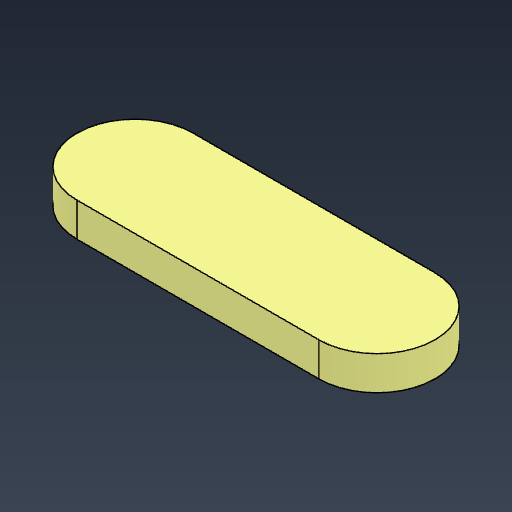
# Autodesk Inventor part: Dribblerdaempfer Unten V2
Saved by Autodesk Inventor 2023.1 (Build 271208000, 208)
## iProperties
Part Number: Dribblerdaempfer Unten V2
Material: Gummi, Silikon
Document SubType Name: Modeling
Designer: rYan
Density: 1.25 g/cm^3
Appearance: Gummi - Schwarz
Mass: 0.126032 g
Surface Area: 3.04725 cm^2
Volume: 0.100826 cm^3
Author: rYan
Autodesk Inventor part; units mm, degrees
ref_plane "YZ Plane" through (0, 0, 0) normal (1, 0, 0) x (0, 1, 0)
ref_plane "XZ Plane" through (0, 0, 0) normal (0, 1, 0) x (-1, 0, 0)
ref_plane "XY Plane" through (0, 0, 0) normal (0, 0, 1) x (1, 0, 0)
sketch "Skizze1" plane through (0, 0, 0) normal (0, 1, 0) x (-1, 0, 0)
  line L0 (0, 0) -> (14.8, 0)
  line L1 (14.8, 0) -> (14.8, 1.4)
  line L2 (0, 1.4) -> (0, 0)
  line L3 (14.8, 1.4) -> (11.5, 1.4)
  line L4 (11.5, 1.4) -> (11.5, 1.4)
  line L5 (11.1, 1.4) -> (11.1, 1.4)
  line L6 (7.6, 1.4) -> (0, 1.4)
  line L7 (11.1, 1.4) -> (8, 1.4)
  line L8 (8, 1.4) -> (8, 1.4)
  line L9 (7.6, 1.4) -> (7.6, 1.4)
  line L10 (11.5, 1.4) -> (11.1, 1.4)
  line L11 (8, 1.4) -> (7.6, 1.4)
  line L12 (11.3, 1.4) -> (11.3, 0.8) construction
  line L13 (7.8, 1.4) -> (7.8, 0.8) construction
  dimension "d1" = 14.8
  dimension "d3" = 1.4
  dimension "d17" = 1.4
  dimension "d18" = 1.4
  dimension "d19" = 3.5
  dimension "d20" = 0.4
  dimension "d21" = 0.4
  dimension "d22" = 7
  dimension "d23" = 60
  dimension "d24" = 60
  constraints: 28 end point, 4 horizontal, 3 point on line, 2 equal length, 2 midpoint, 2 vertical, 1 perpendicular, 2 other
  measures "d1" distance of L0.start L0.end
  measures "d3" distance of L2.start L0.start
  measures "d17" distance between parallel lines of L10 L0
  measures "d18" distance between parallel lines of L11 L0
  measures "d19" distance between parallel lines of L1 L12
  measures "d20" distance of L4.end L5.start
  measures "d21" distance of L8.end L9.start
  measures "d22" distance between parallel lines of L13 L1
  measures "d23" angle of L5 L4
  measures "d24" angle of L9 L8
extrude "Extrusion1" add sketch "Skizze1" along normal mid plane 4.8
fillet "Rundung1" radius 2.4 4 edges at (0, 2.4, 0.7) (-14.8, -2.4, 0.7) (-14.8, 2.4, 0.7) (0, -2.4, 0.7)
equation "\"d24\" = d23"
